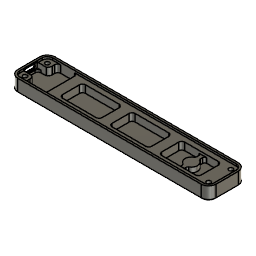
charge_dock_case (Autodesk Fusion 360 design; units mm, degrees)
part number: 2026-08-27-21-34-13-653
part number: 2026-08-29-18-29-15-776
Autodesk Fusion 360 part; units mm, degrees
sketch "PLANNING" plane through (0, 0, 0) normal (0, 0, 1) x (1, 0, 0)
  line L0 (-74, -15) -> (74, -15)
  line L1 (80, -9) -> (80, 9)
  line L2 (74, 15) -> (-74, 15)
  line L3 (-80, 9) -> (-80, -9)
  line L4 (-80, -15) -> (80, 15) construction
  line L5 (80, -15) -> (-80, 15) construction
  arc A0 (-74, 15) -> (-80, 9) centre (-74, 9) ccw
  arc A1 (-80, -9) -> (-74, -15) centre (-74, -9) ccw
  arc A2 (74, -15) -> (80, -9) centre (74, -9) ccw
  arc A3 (80, 9) -> (74, 15) centre (74, 9) ccw
  line L6 (-78, 9) -> (-78, -9)
  arc A4 (-78, -9) -> (-74, -13) centre (-74, -9) ccw
  line L7 (-74, -13) -> (74, -13)
  arc A5 (74, -13) -> (78, -9) centre (74, -9) ccw
  line L8 (78, -9) -> (78, 9)
  arc A6 (78, 9) -> (74, 13) centre (74, 9) ccw
  line L9 (74, 13) -> (-74, 13)
  arc A7 (-74, 13) -> (-78, 9) centre (-74, 9) ccw
  line L10 (0, 0) -> (-50, 0) construction
  line L11 (-49.2929, 2.8284) -> (-52.8284, -0.7071)
  arc A8 (-52.8284, -0.7071) -> (-50.7071, -2.8284) centre (-51.7678, -1.7678) ccw
  line L12 (-50.7071, -2.8284) -> (-47.1716, 0.7071)
  arc A9 (-47.1716, 0.7071) -> (-49.2929, 2.8284) centre (-48.2322, 1.7678) ccw
  line L13 (-48.2322, 1.7678) -> (-51.7678, -1.7678) construction
  line L14 (-10.7071, -2.8284) -> (-7.1716, 0.7071)
  arc A10 (-7.1716, 0.7071) -> (-9.2929, 2.8284) centre (-8.2322, 1.7678) ccw
  arc A11 (-12.8284, -0.7071) -> (-10.7071, -2.8284) centre (-11.7678, -1.7678) ccw
  line L15 (-9.2929, 2.8284) -> (-12.8284, -0.7071)
  line L16 (29.2929, -2.8284) -> (32.8284, 0.7071)
  arc A12 (32.8284, 0.7071) -> (30.7071, 2.8284) centre (31.7678, 1.7678) ccw
  arc A13 (27.1716, -0.7071) -> (29.2929, -2.8284) centre (28.2322, -1.7678) ccw
  line L17 (30.7071, 2.8284) -> (27.1716, -0.7071)
  line L18 (69.2929, -2.8284) -> (72.8284, 0.7071)
  arc A14 (72.8284, 0.7071) -> (70.7071, 2.8284) centre (71.7678, 1.7678) ccw
  arc A15 (67.1716, -0.7071) -> (69.2929, -2.8284) centre (68.2322, -1.7678) ccw
  line L19 (70.7071, 2.8284) -> (67.1716, -0.7071)
  line L20 (-78, 0) -> (-68, 0) construction
  circle A16 centre (-74, 9) radius 1.35
  circle A17 centre (-74, -9) radius 1.35
  line L21 (0, 0) -> (0, -13) construction
  circle A18 centre (74, 9) radius 1.35
  circle A19 centre (74, -9) radius 1.35
  point P0 (-50, 0)
  point P1 (-52.8284, -2.8284)
  point P2 (-47.1716, 2.8284)
  dimension "d1" = 30
  dimension "d2" = 160
  dimension "d3" = 6
  dimension "d4" = -2
  dimension "d5" = 45
  dimension "d7" = 8
  dimension "d8" = 3
  dimension "d11" = 40
  dimension "d12" = 0
  dimension "d13" = 50
  dimension "d14" = 10
  dimension "d15" = 2.7
  constraint horizontal L0
  constraint perpendicular L0 L1
  constraint parallel L0 L2
  constraint parallel L1 L3
  constraint coincident L4 L10.start
  constraint coincident L5 L10.start
  constraint coincident L10.start L21.start
  constraint coincident L5.end L2
  constraint coincident L5.end L3
  constraint tangent L2 A0
  constraint tangent L3 A0
  constraint coincident L4.start L3
  constraint coincident L4.start L0
  constraint tangent L3 A1
  constraint tangent L0 A1
  constraint equal A0 A1
  constraint coincident L5.start L0
  constraint coincident L5.start L1
  constraint tangent L0 A2
  constraint tangent L1 A2
  constraint equal A0 A2
  constraint coincident L4.end L1
  constraint coincident L4.end L2
  constraint tangent L1 A3
  constraint tangent L2 A3
  constraint equal A0 A3
  constraint parallel L2 L10
  constraint tangent L11 A8
  constraint tangent A8 L12
  constraint parallel L11 L12
  constraint tangent L12 A9
  constraint tangent L11 A9
  constraint coincident P0 L10.end
  constraint midpoint L13 P0
  constraint midpoint A8 P1
  constraint midpoint A9 P2
  constraint midpoint L6 L20.start
  constraint perpendicular L6 L20
  constraint concentric A0 A16
  constraint concentric A1 A17
  constraint equal A16 A17
  constraint midpoint L7 L21.end
  constraint perpendicular L7 L21
  constraint symmetric A16 L21 A18
  constraint symmetric A17 L21 A19
  measures "d1" distance of L4.start L5.end
  measures "d2" distance of L4.end L5.end
  measures "d3" radius of A0
  measures "d5" angle of L10 L13
  measures "d7" distance of P1 P2
  measures "d8" distance of L11 L12
  measures "d13" distance of L10.start L10.end
  measures "d14" distance of L20.start L20.end
  measures "d15" diameter of A16
sketch "PCB_REF" plane through (0, 0, 0) normal (0, 0, 1) x (1, 0, 0)
  line L0 (-78, 9) -> (-78, -9)
  arc A0 (-78, -9) -> (-74, -13) centre (-74, -9) ccw
  line L1 (-74, -13) -> (74, -13)
  arc A1 (74, -13) -> (78, -9) centre (74, -9) ccw
  line L2 (78, -9) -> (78, 9)
  arc A2 (78, 9) -> (74, 13) centre (74, 9) ccw
  arc A3 (-74, 13) -> (-78, 9) centre (-74, 9) ccw
  line L3 (74, 13) -> (-74, 13)
  circle A4 centre (-74, 9) radius 1.35
  circle A5 centre (-74, -9) radius 1.35
  line L4 (-49.2929, 2.8284) -> (-52.8284, -0.7071) construction
  arc A6 (-52.8284, -0.7071) -> (-50.7071, -2.8284) centre (-51.7678, -1.7678) ccw construction
  arc A7 (-47.1716, 0.7071) -> (-49.2929, 2.8284) centre (-48.2322, 1.7678) ccw construction
  line L5 (-50.7071, -2.8284) -> (-47.1716, 0.7071) construction
  circle A8 centre (74, 9) radius 1.35
  circle A9 centre (74, -9) radius 1.35
  line L6 (-48.2322, 1.7678) -> (-51.7678, -1.7678)
  line L7 (-51.0607, 1.0607) -> (-48.9393, -1.0607)
  line L8 (-11.0607, 1.0607) -> (-8.9393, -1.0607)
  line L9 (-8.2322, 1.7678) -> (-11.7678, -1.7678)
  line L10 (28.9393, 1.0607) -> (31.0607, -1.0607)
  line L11 (31.7678, 1.7678) -> (28.2322, -1.7678)
  line L12 (68.9393, 1.0607) -> (71.0607, -1.0607)
  line L13 (71.7678, 1.7678) -> (68.2322, -1.7678)
  line L14 (-78, 0) -> (-68, 0)
  dimension "d18" = 40
  dimension "d19" = 0
  constraint coincident A7.centre L6.start
  constraint coincident A6.centre L6.end
  constraint midpoint L4 L7.start
  constraint midpoint L5 L7.end
sketch "Sketch1" plane through (0, 0, 0) normal (0, 0, 1) x (1, 0, 0) in component "Base"
  line L0 (-80, 9) -> (-80, -9)
  arc A0 (-80, -9) -> (-74, -15) centre (-74, -9) ccw
  line L1 (-74, -15) -> (74, -15)
  arc A1 (74, -15) -> (80, -9) centre (74, -9) ccw
  line L2 (80, -9) -> (80, 9)
  arc A2 (80, 9) -> (74, 15) centre (74, 9) ccw
  arc A3 (-74, 15) -> (-80, 9) centre (-74, 9) ccw
  line L3 (74, 15) -> (-74, 15)
  line L4 (-78, 9) -> (-78, -9) construction
  arc A4 (-78, -9) -> (-74, -13) centre (-74, -9) ccw construction
  line L5 (-74, -13) -> (74, -13) construction
  arc A5 (74, -13) -> (78, -9) centre (74, -9) ccw construction
  line L6 (78, -9) -> (78, 9) construction
  arc A6 (78, 9) -> (74, 13) centre (74, 9) ccw construction
  arc A7 (-74, 13) -> (-78, 9) centre (-74, 9) ccw construction
  line L7 (74, 13) -> (-74, 13) construction
  line L8 (-78.3, 9) -> (-78.3, -9)
  arc A8 (-78.3, -9) -> (-74, -13.3) centre (-74, -9) ccw
  line L9 (-74, -13.3) -> (74, -13.3)
  arc A9 (74, -13.3) -> (78.3, -9) centre (74, -9) ccw
  line L10 (78.3, -9) -> (78.3, 9)
  arc A10 (78.3, 9) -> (74, 13.3) centre (74, 9) ccw
  line L11 (74, 13.3) -> (-74, 13.3)
  arc A11 (-74, 13.3) -> (-78.3, 9) centre (-74, 9) ccw
  circle A12 centre (-74, 9) radius 4 construction
  line L12 (-70, 9) -> (-70, 13.3)
  line L13 (-74, 5) -> (-78.3, 5)
  arc A13 (-74, 5) -> (-70, 9) centre (-74, 9) ccw
  line L14 (0, 0) -> (0, -13.3) construction
  line L15 (0, 0) -> (-78.3, 0) construction
  circle A14 centre (-74, 9) radius 1.7
  circle A15 centre (-74, -9) radius 1.7
  line L16 (-74, -5) -> (-78.3, -5)
  arc A16 (-70, -9) -> (-74, -5) centre (-74, -9) ccw
  line L17 (-70, -9) -> (-70, -13.3)
  line L18 (74, 5) -> (78.3, 5)
  arc A17 (70, 9) -> (74, 5) centre (74, 9) ccw
  line L19 (70, 9) -> (70, 13.3)
  circle A18 centre (74, 9) radius 1.7
  line L20 (70, -9) -> (70, -13.3)
  arc A19 (74, -5) -> (70, -9) centre (74, -9) ccw
  line L21 (74, -5) -> (78.3, -5)
  circle A20 centre (74, -9) radius 1.7
  line L22 (-78.3, 5.8) -> (-71.6, 5.8)
  line L23 (-78.3, -5.8) -> (-71.6, -5.8)
  dimension "d22" = 0.3
  dimension "d23" = 3.4
  dimension "d46" = 0.8
  constraint concentric A7 A12
  constraint coincident L4.start A12
  constraint coincident A12 L12.start
  constraint coincident L11 L12.end
  constraint perpendicular L11 L12
  constraint coincident A12 L13.start
  constraint coincident L8 L13.end
  constraint perpendicular L8 L13
  constraint tangent A12 L13
  constraint tangent A12 L12
  constraint tangent L13 A13
  constraint tangent L12 A13
  constraint coincident L14.start L15.start
  constraint midpoint L9 L14.end
  constraint perpendicular L9 L14
  constraint midpoint L8 L15.end
  constraint concentric A7 A14
  constraint symmetric L12.start L15 A16.start
  constraint symmetric L12.end L15 L17.end
  constraint symmetric L13.start L15 L16.start
  constraint symmetric L13.end L15 L16.end
  constraint symmetric A13 L15 A16
  constraint symmetric L15 A14 A15
  constraint symmetric L12.start L14 A17.start
  constraint symmetric L12.end L14 L19.end
  constraint symmetric L13.start L14 L18.start
  constraint symmetric L13.end L14 L18.end
  constraint symmetric A13 L14 A17
  constraint symmetric L14 A14 A18
  constraint symmetric L14 A15 A20
  constraint symmetric L14 L16.start A19.start
  constraint symmetric L14 L16.end L21.end
  constraint symmetric L14 A16.start L20.start
  constraint symmetric L14 A16 A19
  constraint symmetric L14 L17.end L20.end
  constraint coincident L8 L22.start
  constraint coincident A12 L22.end
  constraint perpendicular L4 L22
  constraint symmetric L15 L22.start L23.start
  constraint symmetric L15 L22.end L23.end
  measures "d23" diameter of A14
  measures "d46" distance of L13 L22
extrude "Extrude1" add sketch "Sketch1" along normal blind 1.6 contours L0 A0 L1 A1 L2 A2 A3 L3 in component "Base"
extrude "Extrude2" add sketch "Sketch1" against normal blind 6 contours L0 A0 L1 A1 L2 A2 A3 L3 | L8 L11 A11 L12 A13 L22 | L10 A10 L11 L18 A17 L19 | L8 A8 L9 A16 L17 L23 | L9 A9 L10 L20 A19 L21 in component "Base"
extrude "Extrude3" add sketch "Sketch1" against normal blind 3 from surface at -6 contours L0 A0 L1 A1 L2 A2 A3 L3 | L8 L11 A11 L12 A13 L22 | L8 L13 A13 L22 | L8 L9 L10 L11 L12 L13 A13 L16 A16 L17 L18 A17 L19 L20 A19 L21 | L8 L16 A16 L23 | L10 A10 L11 L18 A17 L19 | L8 A8 L9 A16 L17 L23 | L9 A9 L10 L20 A19 L21 | A14 | A15 | A18 | A20 in component "Base"
sketch "Sketch3" plane through (0, 0, 0) normal (0, 0, 1) x (1, 0, 0) in component "Base"
  line L0 (-74, 13.3) -> (74, 13.3)
  arc A0 (-74, 13.3) -> (-78.3, 9) centre (-74, 9) ccw
  line L1 (-78.3, -9) -> (-78.3, 9)
  arc A1 (-78.3, -9) -> (-74, -13.3) centre (-74, -9) ccw
  line L2 (74, -13.3) -> (-74, -13.3)
  arc A2 (74, -13.3) -> (78.3, -9) centre (74, -9) ccw
  line L3 (78.3, 9) -> (78.3, -9)
  arc A3 (78.3, 9) -> (74, 13.3) centre (74, 9) ccw
  line L4 (-54, 13.3) -> (-54, -13.3)
  line L5 (-46, 13.3) -> (-46, -13.3)
  line L6 (-6, 13.3) -> (-6, -13.3)
  line L7 (-14, 13.3) -> (-14, -13.3)
  line L8 (34, 13.3) -> (34, -13.3)
  line L9 (26, 13.3) -> (26, -13.3)
  line L10 (74, 13.3) -> (74, -13.3) construction
  line L11 (66, 13.3) -> (66, -13.3)
  line L12 (-46, 9.3) -> (66, 9.3)
  line L13 (0, 0) -> (-46, 0) construction
  line L14 (-46, -9.3) -> (66, -9.3)
  line L15 (70, 13.3) -> (70, 9)
  arc A4 (70, 9) -> (74, 5) centre (74, 9) ccw
  line L16 (74, 5) -> (78.3, 5)
  line L17 (78.3, -5) -> (74, -5)
  arc A5 (74, -5) -> (70, -9) centre (74, -9) ccw
  line L18 (70, -9) -> (70, -13.3)
  dimension "d31" = 46
  dimension "d32" = 54
  dimension "d35" = 40
  dimension "d36" = 0
  dimension "d37" = 4
  constraint coincident L0 L4.start
  constraint coincident L2 L4.end
  constraint perpendicular L2 L4
  constraint coincident L0 L5.start
  constraint coincident L2 L5.end
  constraint perpendicular L2 L5
  constraint coincident L5 L12.start
  constraint coincident L11 L12.end
  constraint perpendicular L11 L12
  constraint coincident L13.start origin
  constraint midpoint L5 L13.end
  constraint symmetric L12.start L13 L14.start
  constraint symmetric L12.end L13 L14.end
  measures "d31" distance of L13.start L5
  measures "d32" distance of L13.start L4
  measures "d37" distance of L0 L12
extrude "Extrude4" add sketch "Sketch3" against normal up to surface (6 mm away) contours L0 L2 L4 L5 | L0 L5 L7 L12 | L0 L6 L7 L12 | L2 L5 L7 L14 | L0 L6 L9 L12 | L6 L7 L12 L14 | L2 L6 L7 L14 | L0 L8 L9 L12 | L2 L6 L9 L14 | L0 L8 L11 L12 | L8 L9 L12 L14 | L2 L8 L9 L14 | L0 L2 L3 L11 L15 A4 L16 L17 A5 L18 | L2 L8 L11 L14 in component "Base"
sketch "Sketch4" plane through (-80, 0, 0) normal (-1, 0, 0) x (0, -1, 0) in component "Base"
  line L0 (9, -9) -> (9, 1.6)
  line L1 (9, 1.6) -> (-9, 1.6)
  line L2 (-9, 1.6) -> (-9, -9)
  line L3 (-9, -9) -> (9, -9)
  line L4 (-2.775, -3.35) -> (2.775, -3.35)
  arc A0 (2.775, -3.35) -> (2.775, -0.25) centre (2.775, -1.8) ccw
  line L5 (2.775, -0.25) -> (-2.775, -0.25)
  arc A1 (-2.775, -0.25) -> (-2.775, -3.35) centre (-2.775, -1.8) ccw
  line L6 (-2.775, -1.8) -> (2.775, -1.8) construction
  line L7 (0, -1.8) -> (0, 1.6) construction
  point P0 (0, -1.8)
  point P1 (4.325, -1.8)
  dimension "d41" = 3.4
  dimension "d42" = 3.1
  dimension "d43" = 4.325
  constraint tangent L4 A0
  constraint tangent A0 L5
  constraint parallel L4 L5
  constraint tangent L5 A1
  constraint tangent L4 A1
  constraint parallel L1 L6
  constraint midpoint L6 P0
  constraint coincident P0 L7.start
  constraint midpoint L1 L7.end
  constraint perpendicular L1 L7
  constraint midpoint A0 P1
  measures "d41" distance of P0 L7.end
  measures "d42" distance of L4 L5
  measures "d43" distance of P0 P1
extrude "Extrude5" cut sketch "Sketch4" against normal up to surface (1.7 mm away) contours L4 A0 L5 A1 in component "Base"
chamfer "Chamfer2" distance 1 angle 45 1 faces at (-24.6667, 5, -9) in component "Base"
sketch "Sketch5" plane through (0, 0, -9) normal (0, 0, -1) x (1, 0, 0) in component "Base"
  arc A0 (-79, -9) -> (-74, -14) centre (-74, -9) ccw
  line L0 (-74, -14) -> (74, -14)
  arc A1 (74, -14) -> (79, -9) centre (74, -9) ccw
  line L1 (79, -9) -> (79, 9)
  arc A2 (79, 9) -> (74, 14) centre (74, 9) ccw
  line L2 (74, 14) -> (-74, 14)
  arc A3 (-74, 14) -> (-79, 9) centre (-74, 9) ccw
  line L3 (-79, 9) -> (-79, -9)
  line L4 (0, 0) -> (51, 0) construction
  circle A4 centre (51, 0) radius 2.35
  line L5 (0, 0) -> (0, -14) construction
  circle A5 centre (51, 0) radius 5
  circle A6 centre (-51, 0) radius 2.35
  circle A7 centre (-51, 0) radius 5
  dimension "d48" = 4.7
  dimension "d49" = 10
  dimension "d50" = 102
  constraint coincident L4.start L5.start
  constraint perpendicular L1 L4
  constraint coincident L4.end A4.centre
  constraint midpoint L0 L5.end
  constraint concentric A4 A5
  constraint symmetric A4 L5 A6
  constraint symmetric L5 A5 A7
  measures "d48" diameter of A4
  measures "d49" diameter of A5
  measures "d50" distance of L4.end A6.centre
extrude "Extrude6" add sketch "Sketch5" against normal blind 7 contours A4 | A5 | A6 | A7 in component "Base"
extrude "Extrude7" cut sketch "Sketch5" against normal blind 6 contours A4 | A6 in component "Base"
sketch "Sketch6" plane through (0, 0, 0) normal (0, 0, 1) x (1, 0, 0) in component "Base"
  line L0 (0.5, -29.9958) -> (-0.5, -29.9958)
  line L1 (-0.5, -29.9958) -> (-0.5, 29.9958)
  line L2 (-0.5, 29.9958) -> (0.5, 29.9958)
  line L3 (0.5, 29.9958) -> (0.5, -29.9958)
  line L4 (0.5, -29.9958) -> (-0.5, 29.9958) construction
  line L5 (-0.5, -29.9958) -> (0.5, 29.9958) construction
  line L6 (-60.5, -29.9958) -> (-60.5, 29.9958)
  line L7 (-60.5, 29.9958) -> (-59.5, 29.9958)
  line L8 (-59.5, -29.9958) -> (-60.5, -29.9958)
  line L9 (-59.5, 29.9958) -> (-59.5, -29.9958)
  line L10 (-30.5, -29.9958) -> (-30.5, 29.9958)
  line L11 (-30.5, 29.9958) -> (-29.5, 29.9958)
  line L12 (-29.5, -29.9958) -> (-30.5, -29.9958)
  line L13 (-29.5, 29.9958) -> (-29.5, -29.9958)
  line L14 (29.5, -29.9958) -> (29.5, 29.9958)
  line L15 (29.5, 29.9958) -> (30.5, 29.9958)
  line L16 (30.5, -29.9958) -> (29.5, -29.9958)
  line L17 (30.5, 29.9958) -> (30.5, -29.9958)
  line L18 (59.5, -29.9958) -> (59.5, 29.9958)
  line L19 (59.5, 29.9958) -> (60.5, 29.9958)
  line L20 (60.5, -29.9958) -> (59.5, -29.9958)
  line L21 (60.5, 29.9958) -> (60.5, -29.9958)
  dimension "d56" = 1
  dimension "d57" = 60
  dimension "d60" = 30
  dimension "d61" = 0
  constraint horizontal L0
  constraint perpendicular L0 L1
  constraint parallel L0 L2
  constraint parallel L1 L3
  constraint coincident L4 origin
  constraint coincident L5 origin
  measures "d56" distance of L0.start L0.end
  measures "d57" distance of L0.start L1.end
extrude "Extrude8" cut sketch "Sketch6" along normal blind 0.4 from surface at -9 in component "Base"
extrude "Extrude9" cut sketch "Sketch6" along normal blind 0.8 from surface at -9 contours L10 L11 L12 L13 | L14 L15 L16 L17 in component "Base"
sketch "Sketch7" plane through (0, 0, -2) normal (0, 0, 1) x (-1, 0, 0) in component "Base"
  circle A0 centre (-51, 0) radius 5
  line L0 (-49.5, -9.3) -> (-52.5, -9.3)
  line L1 (-52.5, -9.3) -> (-52.5, 9.3)
  line L2 (-52.5, 9.3) -> (-49.5, 9.3)
  line L3 (-49.5, 9.3) -> (-49.5, -9.3)
  line L4 (-49.5, -9.3) -> (-52.5, 9.3) construction
  line L5 (-52.5, -9.3) -> (-49.5, 9.3) construction
  line L6 (-66, 9.3) -> (-34, 9.3) construction
  point P0 (-51, 0)
  dimension "d70" = 3
  constraint horizontal L0
  constraint perpendicular L0 L1
  constraint parallel L0 L2
  constraint parallel L1 L3
  constraint coincident L4 P0
  constraint coincident L5 P0
  constraint coincident P0 A0.centre
  constraint collinear L2 L6
  measures "d70" distance of L1 L3
extrude "Extrude10" add sketch "Sketch7" against normal up to surface (4 mm away) contours A0 L1 L2 L3 | A0 L0 L1 L3 in component "Base"
fillet "Fillet2" radius 1.6 10 edges at (49.5, 9.3, -4) (49.5, -4.7697, -4) (52.5, 9.3, -4) (52.5, -4.7697, -4) (52.5, -9.3, -4) (52.5, 4.7697, -4) (49.5, -9.3, -4) (49.5, 4.7697, -4) (-54, 4, -4) (-54, -4, -4) in component "Base"
fillet "Fillet2" radius 2.4 18 edges at (66, -9.3, -3) (26, -9.3, -3) (-14, -9.3, -3) (-54, -13.3, -3) (66, 9.3, -3) (26, 9.3, -3) (-14, 9.3, -3) (-54, 13.3, -3) (-46, 9.3, -3) (-6, 9.3, -3) (34, 9.3, -3) (-46, -9.3, -3) (-6, -9.3, -3) (34, -9.3, -3) (-70, 13.3, -3) (-70, -13.3, -3) (-78.3, -5.8, -3) (-78.3, 5.8, -3) in component "Base"
sketch "Sketch8" plane through (0, 0, 0) normal (0, 0, 1) x (-1, 0, 0) in component "Base"
  line L0 (74, 13.3) -> (67.6, 13.3)
  arc A0 (70, 10.9) -> (67.6, 13.3) centre (67.6, 10.9) ccw
  line L1 (70, 10.9) -> (70, 9)
  arc A1 (70, 9) -> (71.6, 5.8) centre (74, 9) ccw
  line L2 (71.6, 5.8) -> (75.9, 5.8)
  arc A2 (78.3, 3.4) -> (75.9, 5.8) centre (75.9, 3.4) ccw
  line L3 (78.3, 3.4) -> (78.3, 9)
  arc A3 (78.3, 9) -> (74, 13.3) centre (74, 9) ccw
  circle A4 centre (74, 9) radius 1.7
  line L4 (75.9, 5.8) -> (78.3, 5.8)
  constraint coincident L2.end A2.end
  constraint coincident L3 L4.end
  constraint tangent A2 L4
extrude "Extrude11" cut sketch "Sketch8" against normal blind 4.2 contours A2 L3 L4 in component "Base"
mirror "Mirror1" about plane through (0, 0, 0) normal (0, 1, 0) of "Extrude11" in component "Base"
sketch "Sketch4 (2)" plane through (-78.3, 0, 0) normal (1, 0, 0) x (0, 1, 0)
  line L0 (5.8, 0) -> (9, 0)
  line L1 (9, 0) -> (9, 1.6)
  line L2 (9, 1.6) -> (-9, 1.6)
  line L3 (-9, 1.6) -> (-9, 0)
  line L4 (-9, 0) -> (-5.8, 0)
  line L5 (-5.8, 0) -> (-5.8, -4.2)
  line L6 (-5.8, -4.2) -> (-3.4, -4.2)
  line L7 (-3.4, -4.2) -> (-3.4, -6)
  line L8 (-3.4, -6) -> (3.4, -6)
  line L9 (3.4, -6) -> (3.4, -4.2)
  line L10 (3.4, -4.2) -> (5.8, -4.2)
  line L11 (5.8, -4.2) -> (5.8, 0)
  arc A0 (2.775, -3.35) -> (2.775, -0.25) centre (2.775, -1.8) ccw construction
  line L12 (2.775, -3.35) -> (-2.775, -3.35)
  arc A1 (-2.775, -0.25) -> (-2.775, -3.35) centre (-2.775, -1.8) ccw construction
  line L13 (-2.775, -0.25) -> (2.775, -0.25)
  line L14 (-5.8, -4.2) -> (5.8, -4.2)
  line L15 (5.8, -4.2) -> (5.8, 0.6)
  line L16 (5.8, 0.6) -> (-5.8, 0.6)
  line L17 (-5.8, 0.6) -> (-5.8, -4.2)
  arc A2 (-2.775, -0.25) -> (-2.775, -3.35) centre (-2.775, -1.8) ccw
  arc A3 (2.775, -3.35) -> (2.775, -0.25) centre (2.775, -1.8) ccw
  line L18 (-2.775, -1.8) -> (2.775, -1.8) construction
  constraint horizontal L14
  constraint vertical L15
  constraint horizontal L16
  constraint vertical L17
  constraint coincident L5.end L6.start
  constraint coincident A1.centre A2.centre
  constraint coincident A0.centre A3.centre
  constraint symmetric L14 L16 L18
  constraint coincident L10.end L11.start
extrude "Extrude12" cut sketch "Sketch4 (2)" against normal up to surface (0.7 mm away) contours L5 L6 L10 L11 L14 L15 L16 L17 in component "Base"
component "Base" placed x (1, 0, 0) y (0, 1, 0) z (0, 0, 1) at (0, 0, 0)
